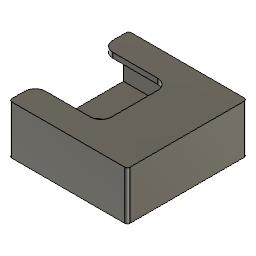
hp48_mount (Autodesk Fusion 360 design; units mm, degrees)
part number: 2026-08-10-19-56-16-923
Autodesk Fusion 360 part; units mm, degrees
sketch "Sketch1" plane through (0, 0, 0) normal (0, 0, 1) x (1, 0, 0)
  line L0 (-28, 37) -> (62, 37)
  line L1 (62, 37) -> (62, 18)
  line L2 (62, 18) -> (-28, 18)
  line L3 (-28, 18) -> (-28, 37)
  dimension "d1" = 90
  dimension "d2" = 19
  constraint horizontal L0
  constraint vertical L1
  constraint horizontal L2
  constraint vertical L3
  measures "d1" distance of L0.start L0.end
  measures "d2" distance of L0.start L2.end
extrude "Extrude1" add sketch "Sketch1" along normal blind 6
sketch "Sketch2" plane through (0, 0, 6) normal (0, 0, 1) x (-1, 0, 0)
  line L0 (28, -37) -> (28, -18)
  line L1 (28, -18) -> (-62, -18)
  line L2 (-62, -18) -> (-62, -37)
  line L3 (-62, -37) -> (28, -37)
ref_plane "WorkPlane1" through (17, 27.5, 6) normal (0, 0, 1) x (-1, 0, 0)
sketch "Sketch3" plane through (0, 0, 6) normal (0, 0, 1) x (1, 0, 0)
  line L0 (17, 37) -> (17, 18)
  circle A0 centre (-8, 27.5) radius 8.9
  circle A1 centre (42, 27.5) radius 8.9
  circle A2 centre (-8, 27.5) radius 3.65
  circle A3 centre (42, 27.5) radius 3.65
  dimension "d13" = 17.8
  dimension "d14" = 17.8
  dimension "d15" = 7.3
  dimension "d16" = 7.3
  constraint vertical L0
  constraint concentric A0 A2
  constraint concentric A1 A3
  measures "d13" diameter of A0
  measures "d14" diameter of A1
  measures "d15" diameter of A2
  measures "d16" diameter of A3
extrude "Extrude2" cut sketch "Sketch3" against normal blind 7 contours A2 | A3
extrude "Extrude3" cut sketch "Sketch3" against normal blind 3
sketch "Sketch4" plane through (0, 0, 0) normal (0, 0, 1) x (1, 0, 0)
  line L0 (-21, 37) -> (55, 37)
  line L1 (55, 37) -> (55, 39)
  line L2 (55, 39) -> (-21, 39)
  line L3 (-21, 39) -> (-21, 37)
  dimension "d21" = 76
  dimension "d22" = 2
  constraint horizontal L0
  constraint vertical L1
  constraint horizontal L2
  constraint vertical L3
  measures "d21" distance of L0.start L0.end
  measures "d22" distance of L0.start L2.end
sketch "Sketch7" plane through (0, 0, 6) normal (0, 0, 1) x (-1, 0, 0)
  circle A0 centre (-42, -27.5) radius 8.9
  circle A1 centre (8, -27.5) radius 8.9
  line L0 (28, -18) -> (-62, -18)
  line L1 (-62, -18) -> (-62, -37)
  line L2 (-62, -37) -> (28, -37)
  line L3 (28, -37) -> (28, -18)
  line L4 (28, -37) -> (-62, -37)
  line L5 (-62, -37) -> (-62, -73)
  line L6 (-62, -73) -> (28, -73)
  line L7 (28, -73) -> (28, -37)
  dimension "d37" = 90
  dimension "d38" = 36
  constraint horizontal L4
  constraint vertical L5
  constraint horizontal L6
  constraint vertical L7
  constraint coincident L2.end L3.start
  measures "d37" distance of L2.end L1.end
  measures "d38" distance of L2.end L6.end
extrude "Extrude7" add sketch "Sketch7" against normal blind 6 contours L2 L4 L5 L6 L7
sketch "Sketch8" plane through (0, 0, 6) normal (0, 0, 1) x (-1, 0, 0)
  circle A0 centre (-42, -27.5) radius 8.9
  circle A1 centre (8, -27.5) radius 8.9
  line L0 (28, -18) -> (-62, -18)
  line L1 (-62, -18) -> (-62, -73)
  line L2 (-62, -73) -> (28, -73)
  line L3 (28, -73) -> (28, -18)
  line L4 (-62, -18) -> (28, -18)
  line L5 (28, -18) -> (28, 18)
  line L6 (28, 18) -> (-62, 18)
  line L7 (-62, 18) -> (-62, -18)
  dimension "d41" = 90
  dimension "d42" = 36
  constraint horizontal L4
  constraint vertical L5
  constraint horizontal L6
  constraint vertical L7
  constraint coincident L0.end L1.start
  measures "d41" distance of L0.end L0.start
  measures "d42" distance of L0.end L6.end
extrude "Extrude8" add sketch "Sketch8" against normal blind 6 contours L0 L4 L5 L6 L7
ref_plane "WorkPlane3" through (17, 27.5, 6) normal (0, 0, 1) x (1, 0, 0)
sketch "Sketch9" plane through (0, 0, 6) normal (0, 0, 1) x (1, 0, 0)
  line L0 (62, -18) -> (-28, -18)
  line L1 (-28, -18) -> (-28, -14)
  line L2 (-28, -14) -> (62, -14)
  line L3 (62, -14) -> (62, -18)
  line L4 (62, 73) -> (-28, 73)
  line L5 (-28, 73) -> (-28, 69)
  line L6 (-28, 69) -> (62, 69)
  line L7 (62, 69) -> (62, 73)
  line L8 (62, -14) -> (62, -14)
  line L9 (62, 69) -> (62, 69)
  line L10 (62, -14) -> (58, -14)
  line L11 (58, -14) -> (58, 69)
  line L12 (58, 69) -> (62, 69)
  line L13 (62, 69) -> (62, -14)
  dimension "d46" = 90
  dimension "d47" = 4
  dimension "d48" = 90
  dimension "d49" = 4
  dimension "d50" = 83
  constraint horizontal L0
  constraint vertical L1
  constraint horizontal L2
  constraint vertical L3
  constraint horizontal L4
  constraint vertical L5
  constraint horizontal L6
  constraint vertical L7
  constraint horizontal L10
  constraint vertical L11
  constraint horizontal L12
  constraint vertical L13
  measures "d46" distance of L0.start L0.end
  measures "d47" distance of L0.start L2.end
  measures "d48" distance of L4.start L4.end
  measures "d49" distance of L4.start L6.end
  measures "d50" distance of L2.end L6.end
extrude "Extrude9" add sketch "Sketch9" along normal blind 27
ref_plane "WorkPlane4" through (17, 27.5, 33) normal (0, 0, 1) x (1, 0, 0)
sketch "Sketch10" plane through (0, 0, 33) normal (0, 0, 1) x (1, 0, 0)
  line L0 (62, -18) -> (22, -18)
  line L1 (22, -18) -> (22, 73)
  line L2 (22, 73) -> (62, 73)
  line L3 (62, 73) -> (62, -18)
  line L4 (62, -18) -> (-28, -18)
  line L5 (-28, -18) -> (-28, 2)
  line L6 (-28, 2) -> (62, 2)
  line L7 (62, 2) -> (62, -18)
  line L8 (62, 73) -> (-28, 73)
  line L9 (-28, 73) -> (-28, 53)
  line L10 (-28, 53) -> (62, 53)
  line L11 (62, 53) -> (62, 73)
  dimension "d54" = 40
  dimension "d55" = 91
  dimension "d56" = 90
  dimension "d57" = 20
  dimension "d58" = 90
  dimension "d59" = 20
  constraint horizontal L0
  constraint vertical L1
  constraint horizontal L2
  constraint vertical L3
  constraint horizontal L4
  constraint vertical L5
  constraint horizontal L6
  constraint vertical L7
  constraint horizontal L8
  constraint vertical L9
  constraint horizontal L10
  constraint vertical L11
  measures "d54" distance of L0.start L0.end
  measures "d55" distance of L0.start L2.end
  measures "d56" distance of L0.start L4.end
  measures "d57" distance of L0.start L6.end
  measures "d58" distance of L2.end L8.end
  measures "d59" distance of L2.end L10.end
extrude "Extrude10" add sketch "Sketch10" along normal blind 4
fillet "Fillet3" radius 8 2 edges at (-28, 2, 35) (-28, 53, 35)
fillet "Fillet4" radius 8 1 edges at (22, 2, 35)
fillet "Fillet5" radius 8 1 edges at (22, 53, 35)
fillet "Fillet6" radius 2 2 edges at (62, -18, 18.5) (-28, -18, 18.5)
fillet "Fillet7" radius 2 7 edges at (-28, 73, 16.5) (-28, 73, 35) (-28, 73, 16.5) (-28, 73, 35) (62, 73, 16.5) (62, 73, 35) (62, 73, 16.5)
